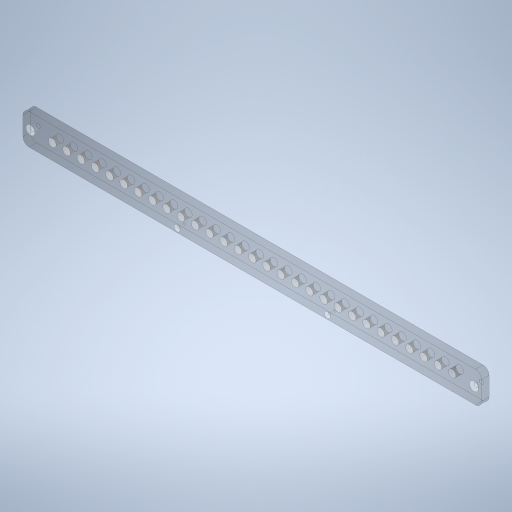
# Autodesk Inventor part: Extremo centella-IN
Saved by Autodesk Inventor 2024.2 (Build 282272000, 272)
## iProperties
Created: 2024-08-26
Part Number: Extremo centella-IN
Material: PMMA Plastic
Document SubType Name: Modeling
Designer: ja.restrepo1
Density: 1.188 g/cm^3
Appearance: Polycarbonate - Clear
Author: ja.restrepo1
Autodesk Inventor part; units mm, degrees
ref_plane "YZ Plane" through (0, 0, 0) normal (1, 0, 0) x (0, 1, 0)
ref_plane "XZ Plane" through (0, 0, 0) normal (0, 1, 0) x (-1, 0, 0)
ref_plane "XY Plane" through (0, 0, 0) normal (0, 0, 1) x (1, 0, 0)
sketch "Sketch1" plane through (0, 0, 0) normal (0, 0, 1) x (1, 0, 0)
  line L0 (-297, 20.5) -> (297, 20.5)
  line L1 (305, 12.5) -> (305, -12.5)
  line L2 (297, -20.5) -> (-297, -20.5)
  line L3 (-305, -12.5) -> (-305, 12.5)
  arc A0 (-297, 20.5) -> (-305, 12.5) centre (-297, 12.5) ccw
  arc A1 (-305, -12.5) -> (-297, -20.5) centre (-297, -12.5) ccw
  arc A2 (305, 12.5) -> (297, 20.5) centre (297, 12.5) ccw
  arc A3 (297, -20.5) -> (305, -12.5) centre (297, -12.5) ccw
  circle A4 centre (266, 0) radius 5
  circle A5 centre (247, 0) radius 5
  circle A6 centre (228, 0) radius 5
  circle A7 centre (209, 0) radius 5
  circle A8 centre (190, 0) radius 5
  circle A9 centre (171, 0) radius 5
  circle A10 centre (152, 0) radius 5
  circle A11 centre (133, 0) radius 5
  circle A12 centre (114, 0) radius 5
  circle A13 centre (95, 0) radius 5
  circle A14 centre (76, 0) radius 5
  circle A15 centre (57, 0) radius 5
  circle A16 centre (38, 0) radius 5
  circle A17 centre (19, 0) radius 5
  circle A18 centre (0, 0) radius 5
  circle A19 centre (-19, 0) radius 5
  circle A20 centre (-38, 0) radius 5
  circle A21 centre (-57, 0) radius 5
  circle A22 centre (-76, 0) radius 5
  circle A23 centre (-95, 0) radius 5
  circle A24 centre (-114, 0) radius 5
  circle A25 centre (-133, 0) radius 5
  circle A26 centre (-152, 0) radius 5
  circle A27 centre (-171, 0) radius 5
  circle A28 centre (-190, 0) radius 5
  circle A29 centre (-209, 0) radius 5
  circle A30 centre (-228, 0) radius 5
  circle A31 centre (-247, 0) radius 5
  circle A32 centre (-266, 0) radius 5
  point P0 (305, -20.5)
  point P1 (305, 20.5)
  point P2 (-305, -20.5)
  point P3 (-305, 0)
  point P4 (0, 20.5)
  point P5 (0, 0)
  dimension "d0" = 610
  dimension "d1" = 41
  dimension "d5" = 8
  dimension "d64" = 10
  dimension "d65" = 39
  dimension "d68" = 19
  constraints: 33 centre point, 8 end point, 8 point on circle, 8 tangent, 6 point on line, 3 equal radius, 2 horizontal, 2 horizontal alignment, 2 midpoint, 2 parallel, 1 perpendicular, 1 vertical alignment, 56 other
  measures "d0" distance of point (305, -20.5) point (-305, -20.5)
  measures "d1" distance of point (305, 20.5) point (305, -20.5)
  measures "d5" radius of A0
  measures "d64" diameter of A4
  measures "d65" distance from line of L1 A4.centre
  measures "d68" distance of A4.centre A5.centre
extrude "Final de centella" add sketch "Sketch1" along normal blind 10
sketch "Sketch2" plane through (0, 0, 10) normal (0, 0, 1) x (1, 0, 0)
  line L0 (-295, 0) -> (295, 0) construction
  line L1 (305, -12.5) -> (305, 12.5) construction
  point P0 (0, 0)
  point P1 (0, 0)
  dimension "d10" = 590
  constraints: 2 coincident, 2 end point, 1 horizontal, 1 midpoint
  measures "d10" distance of L0.start L0.end
hole "Fijación M6" at (-295, 0, 10) at (295, 0, 10) direction (0, 0, -1) diameter 6 end through all countersink diameter 12 countersink angle 90
sketch "Sketch3" plane through (0, 0, 10) normal (0, 0, 1) x (1, 0, 0)
  line L0 (132, 16) -> (266, 16) construction
  line L1 (266, 16) -> (266, -16) construction
  line L2 (305, -12.5) -> (305, 12.5) construction
  line L3 (-21, 16) -> (113, 16) construction
  line L4 (113, 16) -> (113, -16) construction
  line L5 (-174, 16) -> (-40, 16) construction
  line L6 (-40, 16) -> (-40, -16) construction
  line L7 (-325.5, 16) -> (-191.5, 16) construction
  line L8 (-191.5, 16) -> (-191.5, -16) construction
  point P0 (0, 0)
  point P1 (199, -16)
  point P2 (199, 16)
  point P3 (132, -16)
  point P4 (199, 16)
  point P5 (266, 0)
  point P6 (46, -16)
  point P7 (46, 16)
  point P8 (-21, -16)
  point P9 (46, 16)
  point P10 (113, 0)
  point P11 (-107, -16)
  point P12 (-107, 16)
  point P13 (-174, -16)
  point P14 (-107, 16)
  point P15 (-40, 0)
  point P16 (-258.5, -16)
  point P17 (-258.5, 16)
  point P18 (-325.5, -16)
  point P19 (-258.5, 16)
  point P20 (-191.5, 0)
  dimension "d22" = 32
  dimension "d23" = 134
  dimension "d24" = 39
  dimension "d26" = 134
  dimension "d27" = 19
  dimension "d29" = 134
  dimension "d30" = 19
  dimension "d32" = 134
  dimension "d33" = 17.5
  constraints: 20 horizontal alignment, 16 end point, 12 vertical alignment, 8 coincident, 8 midpoint, 4 horizontal, 4 perpendicular, 3 collinear
  measures "d22" distance of L0.end L1.end
  measures "d23" distance of L0.start L0.end
  measures "d24" distance between parallel lines of L2 L1
  measures "d26" distance of L3.start L3.end
  measures "d27" distance of L0.start L3.end
  measures "d29" distance of L5.start L5.end
  measures "d30" distance of L5.end L3.start
  measures "d32" distance of L7.start L7.end
  measures "d33" distance of L5.start L7.end
hole "Fijacion M3 SiPM" [suppressed]
sketch "Sketch6" plane through (0, 0, 10) normal (0, 0, -1) x (-1, 0, 0)
  line L0 (-100, -15.5) -> (100, -15.5) construction
  line L1 (297, -20.5) -> (-297, -20.5) construction
  point P0 (0, 0)
  point P1 (0, -15.5)
  dimension "d73" = 200
  dimension "d74" = 5
  constraints: 2 end point, 1 horizontal, 1 midpoint, 1 vertical alignment
  measures "d73" distance of L0.start L0.end
  measures "d74" distance between parallel lines of L0 L1
hole "Ø4 M4 T madera" at (100, -15.5, 10) at (-100, -15.5, 10) direction (0, 0, -1) diameter 3 end through all countersink diameter 8 countersink angle 90
sketch "Sketch7" plane through (0, 0, 10) normal (0, 0, 1) x (1, 0, 0)
  circle A0 centre (-266, 0) radius 5 projected
  circle A1 centre (-247, 0) radius 5 projected
  circle A2 centre (-228, 0) radius 5 projected
  circle A3 centre (-209, 0) radius 5 projected
  circle A4 centre (-190, 0) radius 5 projected
  circle A5 centre (-171, 0) radius 5 projected
  circle A6 centre (-152, 0) radius 5 projected
  circle A7 centre (-133, 0) radius 5 projected
  circle A8 centre (-114, 0) radius 5 projected
  circle A9 centre (-95, 0) radius 5 projected
  circle A10 centre (-76, 0) radius 5 projected
  circle A11 centre (-57, 0) radius 5 projected
  circle A12 centre (-38, 0) radius 5 projected
  circle A13 centre (-19, 0) radius 5 projected
  circle A14 centre (0, 0) radius 5 projected
  circle A15 centre (19, 0) radius 5 projected
  circle A16 centre (38, 0) radius 5 projected
  circle A17 centre (57, 0) radius 5 projected
  circle A18 centre (76, 0) radius 5 projected
  circle A19 centre (95, 0) radius 5 projected
  circle A20 centre (114, 0) radius 5 projected
  circle A21 centre (133, 0) radius 5 projected
  circle A22 centre (152, 0) radius 5 projected
  circle A23 centre (171, 0) radius 5 projected
  circle A24 centre (190, 0) radius 5 projected
  circle A25 centre (209, 0) radius 5 projected
  circle A26 centre (228, 0) radius 5 projected
  circle A27 centre (247, 0) radius 5 projected
  circle A28 centre (266, 0) radius 5 projected
  point P0 (0, 0)
  constraints: 29 coincident
hole "M12x1.75" at (-266, 0, 10) at (-247, 0, 10) at (-228, 0, 10) at (-209, 0, 10) at (-190, 0, 10) at (-171, 0, 10) at (-152, 0, 10) at (-133, 0, 10) at (-114, 0, 10) at (-95, 0, 10) at (-76, 0, 10) at (-57, 0, 10) at (-38, 0, 10) at (-19, 0, 10) at (0, 0, 10) at (19, 0, 10) at (38, 0, 10) at (57, 0, 10) at (76, 0, 10) at (95, 0, 10) at (114, 0, 10) at (133, 0, 10) at (152, 0, 10) at (171, 0, 10) at (190, 0, 10) at (209, 0, 10) at (228, 0, 10) at (247, 0, 10) at (266, 0, 10) direction (0, 0, -1) diameter 10.106 end through all thread size "M12x1.75" class "6H" standard "ANSI Metric M Profile"
equation "\"d26\" = d23"
equation "\"d29\" = d23"
equation "\"d30\" = d27"
equation "\"d32\" = d23"
body "Solid1"
